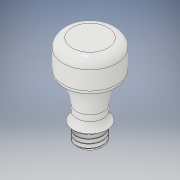
# Autodesk Inventor part: holder
Saved by Autodesk Inventor 2019 (Build 230136000, 136)
## iProperties
Created: 2019-02-19
Part Number: holder
Material: PET Plastic
Document SubType Name: Modeling
Designer: jmc
Density: 1.541 g/cm^3
Appearance: White
Author: jmc
Autodesk Inventor part; units mm, degrees
ref_plane "YZ Plane" through (0, 0, 0) normal (1, 0, 0) x (0, 1, 0)
ref_plane "XZ Plane" through (0, 0, 0) normal (0, 1, 0) x (-1, 0, 0)
sketch "Sketch1" plane through (0, 0, 0) normal (0, 0, 1) x (1, 0, 0)
  line L0 (0, 30) -> (10, 30)
  line L1 (15, 25) -> (15, 14.6932)
  line L2 (7.5, -10) -> (0, -10)
  line L3 (0, 0) -> (15, -30) construction
  line L4 (15, 30) -> (0, 0) construction
  arc A0 (15, 25) -> (10, 30) centre (10, 25) ccw
  arc A1 (14.3935, 12.8658) -> (7.5, -2.1301) centre (27.2577, -2.1301) ccw
  arc A2 (13.5338, 12.0833) -> (15, 14.6932) centre (11.9441, 14.6932) ccw
  line L5 (7.5, -2.1301) -> (7.5, -10)
  line L6 (0, 30) -> (0, -10)
  point P0 (0, 0)
  dimension "d3" = 5
  dimension "d6" = 7.5
  dimension "d57" = 10
  dimension "d62" = 15
  constraints: 15 end point, 8 point on circle, 6 point on line, 4 tangent, 3 centre point, 2 perpendicular, 1 horizontal, 1 parallel, 1 vertical
  measures "d3" radius of A0
  measures "d6" distance of L2.start L2.end
  measures "d57" distance from line of point (0, 0) L2
  measures "d62" distance between parallel lines of L6 L1
revolve "Revolution1" add sketch "Sketch1" angle 360 about axis through (0, 30, 0) along (0, -1, 0) contours L0 A0 L1 A2 A1 L5 L2 L6
sketch "Sketch2" plane through (0, -10, 0) normal (0, -1, 0) x (1, 0, 0)
  circle A0 centre (0, 0) radius 7.5 projected
  circle A1 centre (0, 0) radius 7.5 projected
  point P0 (0, 0)
extrude "Extrusion1" [suppressed]
thread "Thread2" size "5/8-11 UNC" class "2A" standard "ANSI Unified Screw Threads" full length
sketch "Sketch9" plane through (0, -40, 0) normal (-1, 0, 0) x (0, 0, 1)
  line L0 (7.5, 0) -> (7.5, 10)
  line L1 (7.5, 10) -> (5.7879, 10)
  line L2 (5.7879, 10) -> (5.7879, 0)
  line L3 (5.7879, 0) -> (7.5, 0)
  line L4 (0, -2) -> (0, 12) projected
  constraints: 8 end point
revolve "Revolution4" cut sketch "Sketch9" angle 360 about axis through (0, -40, 0) along (0, 1, 0)
sketch "Sketch10" plane through (0, -40, 0) normal (-1, 0, 0) x (0, 0, 1)
  line L0 (7.5, 0) -> (7.5, 10)
  line L1 (7.5, 10) -> (5.7879, 10)
  line L2 (5.7879, 10) -> (5.7879, 0)
  line L3 (5.7879, 0) -> (7.5, 0)
  line L4 (0, -2) -> (0, 12) projected
  constraints: 8 end point
revolve "Revolution5" add sketch "Sketch10" angle 360 about axis through (0, -40, 0) along (0, 1, 0) separate body
sketch "Sketch8" plane through (0, -40, 0) normal (1, 0, 0) x (0, 1, 0)
  line L0 (-1.3471, -5.9048) -> (-1.1546, -5.9048) construction
  line L1 (0.1923, -7.3834) -> (-0.0001, -7.753) construction
  line L2 (-2.3092, -7.753) -> (-2.5016, -7.3834) construction
  line L3 (-0.9622, -5.9048) -> (-1.1546, -5.5352) construction
  line L4 (-1.1546, -5.5352) -> (-1.3471, -5.9048) construction
  line L5 (-2.3092, -7.753) -> (-2.1168, -7.3834) construction
  line L6 (-0.9622, -5.9048) -> (-0.1925, -7.3834)
  line L7 (-2.5016, -7.3834) -> (-2.1168, -7.3834) construction
  arc A0 (-2.5016, -7.3834) -> (-2.3092, -7.5002) centre (-2.3092, -7.2832) ccw construction
  line L8 (0.1923, -7.3834) -> (-0.1925, -7.3834) construction
  line L9 (-2.3092, -7.753) -> (-2.3092, -7.3834) construction
  line L10 (-0.0001, -7.753) -> (-0.0001, -7.3834) construction
  line L11 (-1.1546, -5.5352) -> (-1.1546, -5.7881) construction
  line L12 (-2.3092, -7.5002) -> (-0.0001, -7.5002)
  arc A1 (-2.3092, -7.5002) -> (-2.1168, -7.3834) centre (-2.3092, -7.2832) ccw
  line L13 (-0.1925, -7.3834) -> (-0.0001, -7.753) construction
  line L14 (-2.1168, -7.3834) -> (-1.3471, -5.9048)
  line L15 (-0.0001, -0.0002) -> (-0.0001, 0.0177)
  line L16 (-0.0001, 0.0177) -> (-0.0001, -0.0002)
  line L17 (-0.0001, -0.0002) -> (0.0334, -0.0002)
  arc A2 (-0.1925, -7.3834) -> (-0.0001, -7.5002) centre (-0.0001, -7.2832) ccw
  arc A3 (-0.0001, -7.5002) -> (0.1923, -7.3834) centre (-0.0001, -7.2832) ccw construction
  arc A4 (-1.1546, -5.7881) -> (-1.3471, -5.9048) centre (-1.1546, -6.005) ccw
  arc A5 (-0.9622, -5.9048) -> (-1.1546, -5.7881) centre (-1.1546, -6.005) ccw
  line L18 (-1.1546, -5.7881) -> (-1.1546, -5.9048) construction
  line L19 (-1.1546, -5.9048) -> (-0.9622, -5.9048) construction
  dimension "d35" = 55
  dimension "d36" = 0.3696
  dimension "d37" = 0.3696
  dimension "Sketch8_ThreadOffset" = 0
  dimension "Sketch8_MajorRadius" = 7.5
  dimension "d40" = 2.3091
  dimension "Sketch8_MinorRadius" = 5.7879
  constraints: 40 end point, 12 point on circle, 10 parallel, 8 tangent, 6 centre point, 6 collinear, 2 midpoint, 2 point on line, 1 horizontal, 1 perpendicular, 3 other
  measures "d35" angle of L6 L14
  measures "d36" distance of L3.end L0.end
  measures "d37" distance of L1.end L10.end
  measures "Sketch8_ThreadOffset" distance between parallel lines of L15 L10
  measures "Sketch8_MajorRadius" distance from line of L12 L15.start
  measures "d40" distance from line of L1.end L9
  measures "Sketch8_MinorRadius" distance edge to line of A5 L17
coil "Coil2" sketch "Sketch8" operation cut axis through (0, -40, 0) along (0, 1, 0) pitch 2.3114 turns 6.324384 hand right bodies 2
sketch "Sketch11" plane through (0, -10, 0) normal (0, -1, 0) x (1, 0, 0)
  circle A0 centre (0, 0) radius 6.5
  point P0 (0, 0)
  dimension "d54" = 13
  constraints: 1 centre point, 1 coincident
  measures "d54" diameter of A0
extrude "Extrusion3" add sketch "Sketch11" along normal blind 10 bodies 1
move or copy body "Move Body1" bodies to move or copy 2 copy no translate (0, 20, 0)
ref_plane "Work Plane1" through (0, -10, 0) normal (0, -1, 0) x (1, 0, 0)
ref_plane "Work Plane2" through (0, -5, 0) normal (0, -1, 0) x (1, 0, 0)
sketch "Sketch15" plane through (0, 0, 0) normal (0, 0, 1) x (1, 0, 0)
  line L0 (7.5, -2.1301) -> (7.5, -10) projected
  arc A0 (7.5, -5.4046) -> (9.5, -10) centre (13.7794, -5.4046) ccw
  line L1 (7.5, -5.4046) -> (7.5, -10)
  line L2 (-7.5, -10) -> (7.5, -10) projected
  line L3 (7.5, -10) -> (9.5, -10)
  line L4 (0, -30.9236) -> (0, 40.1539) projected
  point P0 (0, 0)
  constraints: 4 end point, 3 point on circle, 2 collinear, 1 centre point, 1 point on line, 1 tangent
revolve "Revolution6" add sketch "Sketch15" angle 360 about axis through (0, -10, 0) along (0, 1, 0) bodies 1
equation "\"d35\" = d42"
equation "\"d36\" = 0.160083 * Sketch8_Pitch"
equation "\"d37\" = 0.160083 * Sketch8_Pitch"
equation "\"d40\" = Sketch8_Pitch"
equation "\"d18\" = 55deg"
equation "\"Sketch4_Pitch\" = 2.30909"
equation "\"d42\" = 55deg"
equation "\"Sketch8_Pitch\" = 2.30909"
body "Solid1"
body "Solid2"
body "Solid4"
